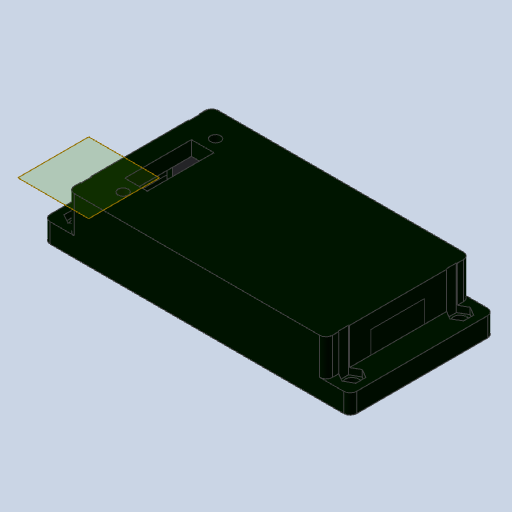
# Autodesk Inventor part: akkum_holder_up
Saved by Autodesk Inventor 2022 (Build 260153000, 153)
## iProperties
Created: 2022-07-21
Part Number: akkum_holder_up
Material: Типовые
Document SubType Name: Modeling
Designer: akapu
Density: 1 g/cm^3
Appearance: По умолчанию
Author: akapu
Autodesk Inventor part; units mm, degrees
ref_plane "YZ Plane" through (0, 0, 0) normal (1, 0, 0) x (0, 1, 0)
ref_plane "XZ Plane" through (0, 0, 0) normal (0, 1, 0) x (-1, 0, 0)
ref_plane "XY Plane" through (0, 0, 0) normal (0, 0, 1) x (1, 0, 0)
sketch "Эскиз1" plane through (0, 0, 0) normal (0, 1, 0) x (-1, 0, 0)
  line L0 (0, 0) -> (-75.2, 0)
  line L1 (-75.2, 0) -> (-75.2, -36.7)
  line L2 (-75.2, -36.7) -> (0, -36.7)
  line L3 (0, -36.7) -> (0, 0)
  line L4 (0, 0) -> (10, 0)
  line L5 (10, 0) -> (10, 4)
  line L6 (10, 4) -> (0, 4)
  line L7 (0, 4) -> (0, 0)
  line L8 (10, 4) -> (-85.2, 4)
  line L9 (-85.2, 4) -> (-85.2, -40.7)
  line L10 (-85.2, -40.7) -> (10, -40.7)
  line L11 (10, -40.7) -> (10, 4)
  line L12 (-75.2, -36.7) -> (-80.2, -36.7)
  line L13 (-80.2, -36.7) -> (-80.2, 0)
  line L14 (-80.2, 0) -> (5, 0)
  line L15 (5, 0) -> (5, -36.7)
  line L16 (5, -36.7) -> (-80.2, -36.7)
  line L17 (-80.2, -36.7) -> (-80.2, -35.1)
  line L18 (-80.2, -35.1) -> (5, -35.1)
  line L19 (5, 0) -> (5, -1.6)
  line L20 (5, -1.6) -> (-80.2, -1.6)
  circle A0 centre (-80.2, -1.6) radius 1.6
  circle A1 centre (-80.2, -35.1) radius 1.6
  circle A2 centre (5, -35.1) radius 1.6
  circle A3 centre (5, -1.6) radius 1.6
  line L21 (5, -1.6) -> (2.4, -1.6)
  line L22 (2.4, -1.6) -> (2.4, -35.1)
  line L23 (-80.2, -1.6) -> (-77.6, -1.6)
  line L24 (-77.6, -1.6) -> (-77.6, -35.1)
  circle A4 centre (5, -1.6) radius 2.05
  circle A5 centre (5, -35.1) radius 2.05
  circle A6 centre (-80.2, -35.1) radius 2.05
  circle A7 centre (-80.2, -1.6) radius 2.05
  dimension "d0" = 75.2
  dimension "d1" = 36.7
  dimension "d2" = 10
  dimension "d3" = 4
  dimension "d4" = 95.2
  dimension "d5" = 44.7
  dimension "d6" = 5
  dimension "d7" = 85.2
  dimension "d8" = 1.6
  dimension "d9" = 1.6
  dimension "d10" = 2.6
  dimension "d11" = 2.6
  dimension "d12" = 4.1
  dimension "d13" = 4.1
  dimension "d14" = 4.1
  dimension "d15" = 4.1
  constraints: 50 end point, 9 point on line, 8 coincident, 8 perpendicular, 7 parallel, 4 centre point, 4 horizontal, 4 vertical alignment, 1 collinear, 1 midpoint, 8 other
  measures "d0" distance of L2.end L1.end
  measures "d1" distance of L1.end L0.end
  measures "d2" distance of L6.end L5.end
  measures "d3" distance of L5.end L4.end
  measures "d4" distance of L10.end L9.end
  measures "d5" distance of L9.end L8.end
  measures "d6" distance of L1.end L12.end
  measures "d7" distance of L13.end L14.end
  measures "d8" distance of L12.end L17.end
  measures "d9" distance of L14.end L19.end
  measures "d10" distance of L21.start L21.end
  measures "d11" distance of L23.start L23.end
  measures "d12" diameter of A4
  measures "d13" diameter of A5
  measures "d14" diameter of A6
  measures "d15" diameter of A7
extrude "Выдавливание1" add sketch "Эскиз1" along normal blind 6 contours L4 A4 L20 L3 | L7 L6 L5 L4 A4 | L0 L14 A7 L13 A6 L12 L2 L16 A5 L15 A4 L4 L11 L10 L9 L8 L7 | L1 L20 A7 L14 | L20 L22 L18 L3 | L1 L18 L24 L20 | L18 A5 L16 L3 | L20 A4 L15 A5 L18 L22 | L1 L12 A6 L18 | L24 L18 A6 L13 A7 L20
sketch "Эскиз3" plane through (0, 0, 0) normal (0, -1, 0) x (1, 0, 0)
  circle A0 centre (-5, -1.6) radius 2.05 projected
  circle A1 centre (-5, -1.6) radius 1.6
  circle A2 centre (-5, -35.1) radius 2.05 projected
  circle A3 centre (-5, -35.1) radius 1.6
  circle A4 centre (80.2, -35.1) radius 2.05 projected
  circle A5 centre (80.2, -35.1) radius 1.6
  circle A6 centre (80.2, -1.6) radius 2.05 projected
  circle A7 centre (80.2, -1.6) radius 1.6
  line L0 (85.2, -40.7) -> (-10, -40.7) projected
  line L1 (-10, 4) -> (85.2, 4) projected
  line L2 (85.2, -40.7) -> (-10, -40.7)
  line L3 (-10, -40.7) -> (-10, 4)
  line L4 (-10, 4) -> (85.2, 4)
  line L5 (85.2, 4) -> (85.2, -40.7)
  line L6 (0, 0) -> (0, -36.7) projected
  line L7 (0, -36.7) -> (75.2, -36.7) projected
  line L8 (0, 0) -> (75.2, 0)
  line L9 (75.2, 0) -> (75.2, -36.7)
  line L10 (75.2, -36.7) -> (0, -36.7)
  line L11 (0, -36.7) -> (0, 0)
  dimension "d18" = 3.2
  dimension "d19" = 3.2
  dimension "d20" = 3.2
  dimension "d21" = 3.2
  constraints: 16 end point, 4 centre point, 4 coincident, 4 parallel, 2 horizontal, 2 perpendicular
  measures "d18" diameter of A1
  measures "d19" diameter of A3
  measures "d20" diameter of A5
  measures "d21" diameter of A7
extrude "Выдавливание2" add sketch "Эскиз3" against normal blind 2 contours A0 | A2 | A4 | A6 | L0 L3 L1 L5
sketch "Эскиз4" plane through (0, 6, 0) normal (0, 1, 0) x (1, 0, 0)
  line L0 (0, 0) -> (-2.5, 0)
  line L1 (-2.5, 0) -> (-2.5, 40.7)
  line L2 (85.2, 40.7) -> (-10, 40.7) projected
  line L3 (75.2, 0) -> (0, 0) projected
  line L4 (75.2, 0) -> (77.7, 0)
  line L5 (77.7, 0) -> (77.7, -4)
  line L6 (-10, -4) -> (85.2, -4) projected
  line L7 (-2.5, 40.7) -> (77.7, 40.7)
  line L8 (77.7, 40.7) -> (77.7, -4)
  line L9 (77.7, -4) -> (-2.5, -4)
  line L10 (-2.5, -4) -> (-2.5, 40.7)
  line L11 (0, 0) -> (0, 36.7) projected
  line L12 (75.2, 36.7) -> (75.2, 0) projected
  line L13 (0, 36.7) -> (75.2, 36.7)
  line L14 (75.2, 36.7) -> (75.2, 0)
  line L15 (75.2, 0) -> (0, 0)
  line L16 (0, 0) -> (0, 36.7)
  dimension "d24" = 2.5
  dimension "d25" = 2.5
  constraints: 24 end point, 4 parallel, 3 horizontal, 3 perpendicular, 3 point on line, 1 vertical
  measures "d24" distance of L0.start L0.end
  measures "d25" distance of L3.start L4.end
extrude "Выдавливание3" add sketch "Эскиз4" along normal blind 6.827 contours L3 L4 L5 L6 L10 L0 | L0 L1 L2 L8 L4 L12 L13 L11
fillet "Сопряжение1" radius 2 8 edges at (77.7, 9.4135, -40.7) (77.7, 9.4135, 4) (-2.5, 9.4135, 4) (-2.5, 9.4135, -40.7) (-10, 3, 4) (85.2, 3, 4) (85.2, 3, -40.7) (-10, 3, -40.7)
ref_plane "РабПлоскость1" through (0, 19.827, 0) normal (0, -1, 0) x (1, 0, 0)
sketch "Эскиз7" plane through (0, 0, 0) normal (0, -1, 0) x (1, 0, 0)
  line L0 (0, 0) -> (0, -36.7) projected
  line L1 (75.2, -36.7) -> (75.2, 0) projected
  line L2 (0, 0) -> (75.2, 0)
  line L3 (75.2, 0) -> (75.2, -36.7)
  line L4 (75.2, -36.7) -> (0, -36.7)
  line L5 (0, -36.7) -> (0, 0)
  line L6 (0, 0) -> (-0.4, 0)
  line L7 (-0.4, 0) -> (75.6, 0)
  line L8 (75.6, 0) -> (75.6, -36.6)
  line L9 (75.6, -36.6) -> (-0.4, -36.6)
  line L10 (-0.4, -36.6) -> (-0.4, 0)
  line L11 (-0.7, 0.3) -> (75.9, 0.3)
  line L12 (75.9, 0.3) -> (75.9, -36.9)
  line L13 (75.9, -36.9) -> (-0.7, -36.9)
  line L14 (-0.7, -36.9) -> (-0.7, 0.3)
  point P0 (75.2, -36.6)
  point P1 (0, -36.6)
  point P2 (75.2, -36.6)
  dimension "d37" = 0.4
  dimension "d38" = 76
  dimension "d73" = 0.3
  constraints: 26 end point, 6 parallel, 4 perpendicular, 2 horizontal, 3 other
  measures "d37" distance of L0.start L6.end
  measures "d38" distance of L8.end L9.end
  measures "d73" distance between parallel lines of L10 L14
extrude "Выдавливание6" cut sketch "Эскиз7" against normal blind 25.827 contours L2 L1 L9 L0 | L0 L9 L10 L6 | L7 L8 L9 L1 | L11 L12 L13 L14
sketch "Эскиз8" plane through (0, 0, 0) normal (0, -1, 0) x (1, 0, 0)
  line L0 (-0.4, 0) -> (75.6, 0) projected
  line L1 (-0.4, 0) -> (-0.4, -10)
  line L2 (-0.4, -36.6) -> (-0.4, 0) projected
  line L3 (0, -36.7) -> (75.2, -36.7) projected
  line L4 (-0.4, -36.7) -> (-0.4, -26.7)
  line L5 (-0.4, -26.7) -> (-2.4, -26.7)
  line L6 (-2.4, -26.7) -> (-2.4, -10)
  line L7 (-2.4, -10) -> (-0.4, -10)
  line L8 (-0.4, -10) -> (-0.4, -26.7)
  line L9 (-2.4, -10) -> (77.6, -10)
  line L10 (77.6, -10) -> (77.6, -26.7)
  line L11 (77.6, -26.7) -> (-2.4, -26.7)
  line L12 (-2.4, -26.7) -> (-2.4, -10)
  point P0 (0, 0)
  point P1 (75.6, -36.7)
  dimension "d41" = 10
  dimension "d42" = 10
  dimension "d43" = 2
  dimension "d44" = 80
  constraints: 20 end point, 4 parallel, 3 point on line, 2 horizontal, 2 perpendicular
  measures "d41" distance of L0.start L1.end
  measures "d42" distance of L4.start L4.end
  measures "d43" distance of L6.end L7.end
  measures "d44" distance of L10.end L11.end
extrude "Выдавливание7" cut sketch "Эскиз8" against normal blind 25.827
sketch "Эскиз9" plane through (0, 12.827, 0) normal (0, 1, 0) x (1, 0, 0)
  line L0 (-0.4, 10) -> (-0.4, 0) projected
  line L1 (0, 36.7) -> (75.2, 36.7) projected
  line L2 (-0.4, 0) -> (75.6, 0)
  line L3 (75.6, 0) -> (75.6, 36.7)
  line L4 (75.6, 36.7) -> (-0.4, 36.7)
  line L5 (-0.4, 36.7) -> (-0.4, 0)
  arc A0 (77.7, 38.7) -> (75.7, 40.7) centre (75.7, 38.7) ccw projected
  line L6 (83.2, 40.7) -> (75.7, 40.7) projected
  line L7 (77.7, 38.7) -> (75.7, 38.7)
  line L8 (75.7, 38.7) -> (75.7, 40.7)
  line L9 (75.7, 40.7) -> (77.7, 40.7)
  line L10 (77.7, 40.7) -> (77.7, 38.7)
  arc A1 (-2.5, -2) -> (-0.5, -4) centre (-0.5, -2) ccw projected
  line L11 (-0.5, -4) -> (75.7, -4) projected
  line L12 (-2.5, -2) -> (-0.5, -2)
  line L13 (-0.5, -2) -> (-0.5, -4)
  line L14 (-0.5, -4) -> (-2.5, -4)
  line L15 (-2.5, -4) -> (-2.5, -2)
  line L16 (-2.5, -4) -> (77.7, -4)
  line L17 (77.7, -4) -> (77.7, 40.7)
  line L18 (77.7, 40.7) -> (-2.5, 40.7)
  line L19 (-2.5, 40.7) -> (-2.5, -4)
  point P0 (0, 0)
  point P1 (-2.5, -2)
  constraints: 32 end point, 8 parallel, 4 horizontal, 4 perpendicular
extrude "Выдавливание8" add sketch "Эскиз9" along normal blind 3 contours L5 L4 L1 L3 L2 L0 | L7 L8 A0 | L17 L16 L11 L13 L12 L19 L18 L8 L7 | L12 L13 A1
sketch "Эскиз10" plane through (0, 12.827, 0) normal (0, -1, 0) x (1, 0, 0)
  line L0 (6.7, -8) -> (6.7, -4)
  line L1 (6.7, -4) -> (6.7, -32.7)
  circle A0 centre (6.7, -4) radius 1.6
  circle A1 centre (6.7, -32.7) radius 1.6
  line L2 (6.7, -32.7) -> (6.7, -4)
  point P0 (0, 0)
  dimension "d50" = 4
  dimension "d51" = 28.7
  constraints: 6 end point, 2 centre point, 2 coincident, 1 point on line, 1 vertical
  measures "d50" distance of L0.start L0.end
  measures "d51" distance of L0.end L1.end
extrude "Выдавливание9" cut sketch "Эскиз10" against normal blind 8
chamfer "Фаска1" distance 2 angle 45 2 edges at (5.1, 12.827, -4) (5.1, 12.827, -32.7)
fillet "Сопряжение2" radius 2 2 edges at (-2.5, 14.327, -40.7) (77.7, 14.327, 4)
sketch "Эскиз11" plane through (0, 15.827, 0) normal (0, 1, 0) x (1, 0, 0)
  arc A0 (-2.5, -2) -> (-0.5, -4) centre (-0.5, -2) ccw projected
  line L0 (-2.5, -2) -> (-0.5, -2)
  line L1 (-0.5, -2) -> (-0.5, -4)
  line L2 (-0.5, -4) -> (-2.5, -4)
  line L3 (-2.5, -4) -> (-2.5, -2)
  line L4 (-2.5, 38.7) -> (-2.5, -2) projected
  line L5 (83.2, 40.7) -> (-8, 40.7) projected
  line L6 (-2.5, 38.7) -> (0, 38.7)
  line L7 (0, 38.7) -> (0, 40.7)
  line L8 (0, 40.7) -> (-2.5, 40.7)
  line L9 (-2.5, 40.7) -> (-2.5, 38.7)
  arc A1 (77.7, 38.7) -> (75.7, 40.7) centre (75.7, 38.7) ccw projected
  line L10 (77.7, 38.7) -> (75.7, 38.7)
  line L11 (75.7, 38.7) -> (75.7, 40.7)
  line L12 (75.7, 40.7) -> (77.7, 40.7)
  line L13 (77.7, 40.7) -> (77.7, 38.7)
  line L14 (77.7, -2) -> (77.7, 38.7) projected
  arc A2 (75.7, -4) -> (77.7, -2) centre (75.7, -2) ccw projected
  line L15 (77.7, -2) -> (75.7, -2)
  line L16 (75.7, -2) -> (75.7, -4)
  line L17 (75.7, -4) -> (77.7, -4)
  line L18 (77.7, -4) -> (77.7, -2)
  line L19 (-2.5, -4) -> (77.7, -4)
  line L20 (77.7, -4) -> (77.7, 40.7)
  line L21 (77.7, 40.7) -> (-2.5, 40.7)
  line L22 (-2.5, 40.7) -> (-2.5, -4)
  point P0 (0, 0)
  point P1 (-0.5, -4)
  constraints: 40 end point, 10 parallel, 5 horizontal, 5 perpendicular, 1 point on line
extrude "Выдавливание10" add sketch "Эскиз11" along normal blind 1.5 contours L0 L1 A0 | L4 L6 L7 L5 L11 L10 L14 L15 L16 L19 L1 L0 | L9 L5 L7 L6 | L16 L15 A2 | L10 L11 A1
fillet "Сопряжение3" radius 2 1 edges at (-2.5, 16.577, -40.7)
sketch "Эскиз6" plane through (0, 19.827, 0) normal (0, -1, 0) x (1, 0, 0)
  line L0 (0, 0) -> (0, -36.7)
  line L1 (0, 0) -> (0, -8)
  line L2 (0, -36.7) -> (75.2, -36.7)
  line L3 (0, -36.7) -> (0, -28.7)
  line L4 (0, -28.7) -> (3.2, -28.7)
  line L5 (3.2, -28.7) -> (10.2, -28.7)
  line L6 (10.2, -28.7) -> (10.2, -8)
  line L7 (10.2, -8) -> (3.2, -8)
  line L8 (3.2, -8) -> (3.2, -28.7)
  dimension "d31" = 8
  dimension "d32" = 8
  dimension "d33" = 3.2
  dimension "d34" = 7
  constraints: 18 end point, 3 point on line
  measures "d31" distance of L0.start L1.end
  measures "d32" distance of L0.end L3.end
  measures "d33" distance of L3.end L4.end
  measures "d34" distance of L4.end L5.end
extrude "Выдавливание5" cut sketch "Эскиз6" along normal blind 8
sketch "Эскиз12" plane through (0, 12.827, 0) normal (0, -1, 0) x (1, 0, 0)
  circle A0 centre (6.7, -32.7) radius 1.6 projected
  circle A1 centre (6.7, -32.7) radius 1.6
  circle A2 centre (6.7, -4) radius 1.6 projected
  circle A3 centre (6.7, -4) radius 1.6
  point P0 (0, 0)
  constraints: 2 centre point, 2 coincident
extrude "Выдавливание11" cut sketch "Эскиз12" against normal blind 8
sketch "Эскиз13" plane through (0, 6, 0) normal (0, 1, 0) x (1, 0, 0)
  circle A0 centre (-5, 1.6) radius 2.05 projected
  line L0 (-5, 1.6) -> (-2.3, 1.6)
  circle A1 centre (-5, 35.1) radius 1.6 projected
  line L1 (-5, 35.1) -> (-2.3, 35.1)
  circle A2 centre (80.2, 35.1) radius 2.05 projected
  line L2 (80.2, 35.1) -> (77.5, 35.1)
  circle A3 centre (80.2, 1.6) radius 2.05 projected
  line L3 (80.2, 1.6) -> (77.5, 1.6)
  line L4 (77.7, -2) -> (77.7, 38.7) projected
  line L5 (77.5, 3.1588) -> (80.2, 4.7177)
  line L6 (80.2, 4.7177) -> (82.9, 3.1588)
  line L7 (82.9, 3.1588) -> (82.9, 0.0412)
  line L8 (82.9, 0.0412) -> (80.2, -1.5177)
  line L9 (80.2, -1.5177) -> (77.5, 0.0412)
  line L10 (77.5, 0.0412) -> (77.5, 3.1588)
  circle A4 centre (80.2, 35.1) radius 1.6 projected
  line L11 (77.5, 36.6588) -> (80.2, 38.2177)
  line L12 (80.2, 38.2177) -> (82.9, 36.6588)
  line L13 (82.9, 36.6588) -> (82.9, 33.5412)
  line L14 (82.9, 33.5412) -> (80.2, 31.9823)
  line L15 (80.2, 31.9823) -> (77.5, 33.5412)
  line L16 (77.5, 33.5412) -> (77.5, 36.6588)
  line L17 (-2.3, 33.5412) -> (-5, 31.9823)
  line L18 (-5, 31.9823) -> (-7.7, 33.5412)
  line L19 (-7.7, 33.5412) -> (-7.7, 36.6588)
  line L20 (-7.7, 36.6588) -> (-5, 38.2177)
  line L21 (-5, 38.2177) -> (-2.3, 36.6588)
  line L22 (-2.3, 36.6588) -> (-2.3, 33.5412)
  line L23 (-2.3, 0.0412) -> (-5, -1.5177)
  line L24 (-5, -1.5177) -> (-7.7, 0.0412)
  line L25 (-7.7, 0.0412) -> (-7.7, 3.1588)
  line L26 (-7.7, 3.1588) -> (-5, 4.7177)
  line L27 (-5, 4.7177) -> (-2.3, 3.1588)
  line L28 (-2.3, 3.1588) -> (-2.3, 0.0412)
  point P0 (0, 0)
  dimension "d67" = 2.7
  dimension "d68" = 2.7
  constraints: 56 end point, 4 coincident, 4 midpoint, 3 horizontal, 1 perpendicular, 52 other
  measures "d67" distance of L0.start L0.end
  measures "d68" distance of L2.start L2.end
extrude "Выдавливание12" cut sketch "Эскиз13" along normal blind 25 and the other way blind 2 contours A0 | A1 | A2 | L4 L15 L16 L2 | L4 L11 L12 L13 L14 L15 | L2 L16 L11 L4 | A3 | L4 L9 L10 L3 | L4 L5 L6 L7 L8 L9 | L3 L10 L5 L4 | A4 | L17 L18 L19 L20 L21 L22 | L23 L24 L25 L26 L27 L28
